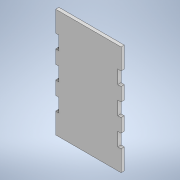
# Autodesk Inventor part: Frontandback_2
Saved by Autodesk Inventor 2020 (Build 240168000, 168)
## iProperties
Created: 2020-12-28
Part Number: Frontandback_2
Material: Generic
Document SubType Name: Modeling
Designer: solar
Density: 1 g/cm^3
Appearance: Default
Author: solar
Autodesk Inventor part; units mm, degrees
ref_plane "YZ Plane" through (0, 0, 0) normal (1, 0, 0) x (0, 1, 0)
ref_plane "XZ Plane" through (0, 0, 0) normal (0, 1, 0) x (-1, 0, 0)
ref_plane "XY Plane" through (0, 0, 0) normal (0, 0, 1) x (1, 0, 0)
sketch "Sketch1" plane through (0, 0, 0) normal (0, 0, 1) x (1, 0, 0)
  line L0 (60, -100) -> (-60, -100)
  line L1 (-60, -100) -> (-60, 100)
  line L2 (-60, 100) -> (60, 100)
  line L3 (60, 100) -> (60, -100)
  line L4 (60, -100) -> (-60, 100) construction
  line L5 (-60, -100) -> (60, 100) construction
  line L6 (60, 0) -> (60, 12.375)
  line L7 (60, 12.375) -> (54, 12.375)
  line L8 (54, 12.375) -> (54, -12.375)
  line L9 (54, -12.375) -> (60, -12.375)
  line L10 (60, 12.375) -> (60, 37.125)
  line L11 (60, 37.125) -> (54, 37.125)
  line L12 (54, 37.125) -> (54, 61.875)
  line L13 (54, 61.875) -> (60, 61.875)
  line L14 (60, -12.375) -> (60, -37.125)
  line L15 (60, -37.125) -> (54, -37.125)
  line L16 (54, -37.125) -> (54, -61.875)
  line L17 (54, -61.875) -> (60, -61.875)
  line L18 (0, 0) -> (0, 100)
  line L19 (0, 0) -> (15.8208, 0)
  line L20 (-60, 12.375) -> (-54, 12.375)
  line L21 (-54, 12.375) -> (-54, -12.375)
  line L22 (-54, -12.375) -> (-60, -12.375)
  line L23 (-60, 37.125) -> (-54, 37.125)
  line L24 (-54, 37.125) -> (-54, 61.875)
  line L25 (-54, 61.875) -> (-60, 61.875)
  line L26 (-60, -37.125) -> (-54, -37.125)
  line L27 (-54, -37.125) -> (-54, -61.875)
  line L28 (-54, -61.875) -> (-60, -61.875)
  dimension "d18" = 120
  dimension "d19" = 200
  dimension "d20" = 12.375
  dimension "d21" = 6
  dimension "d22" = 24.75
  dimension "d23" = 24.75
  dimension "d24" = 6
  dimension "d25" = 24.75
  dimension "d26" = 24.75
  dimension "d27" = 6
  dimension "d28" = 24.75
  constraints: 56 end point, 12 symmetric about line, 7 perpendicular, 5 horizontal, 3 midpoint, 1 parallel, 1 vertical, 10 other
  measures "d18" distance of L1.end L2.end
  measures "d19" distance of L0.end L1.end
  measures "d20" distance of L6.start L6.end
  measures "d21" distance of L6.end L7.end
  measures "d22" distance of L7.end L8.end
  measures "d23" distance of L6.end L10.end
  measures "d24" distance of L10.end L11.end
  measures "d25" distance of L11.end L12.end
  measures "d26" distance of L9.end L14.end
  measures "d27" distance of L14.end L15.end
  measures "d28" distance of L15.end L16.end
extrude "Extrusion1" add sketch "Sketch1" along normal blind 6 contours L0 L1 L28 L27 L26 L22 L21 L20 L23 L24 L25 L2 L3 L13 L12 L11 L7 L8 L9 L15 L16 L17
body "Solid1"
